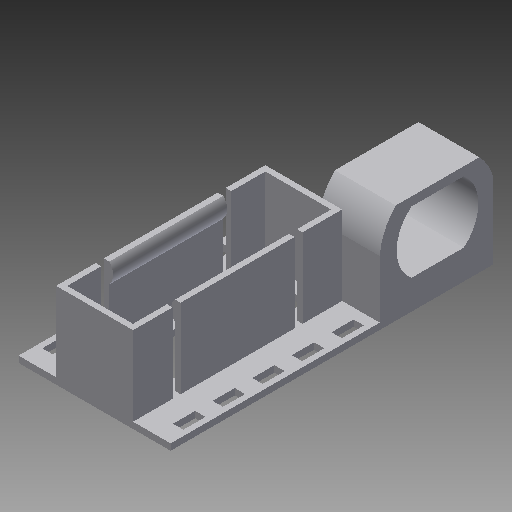
# Autodesk Inventor part: Correct Motor Housing
Saved by Autodesk Inventor 2018 (Build 220112000, 112)
## iProperties
Created: 2014-10-09
Part Number: Correct Motor Housing
Material: Generic
Document SubType Name: Modeling
Designer: Justin
Density: 1 g/cm^3
Appearance: Default(2)
Mass: 11.5799 g
Surface Area: 123.279 cm^2
Volume: 11.5799 cm^3
Author: Justin
Autodesk Inventor part; units mm, degrees
ref_plane "YZ Plane" through (0, 0, 0) normal (1, 0, 0) x (0, 1, 0)
ref_plane "XZ Plane" through (0, 0, 0) normal (0, 1, 0) x (-1, 0, 0)
ref_plane "XY Plane" through (0, 0, 0) normal (0, 0, 1) x (1, 0, 0)
sketch "Sketch1" plane through (0, 0, 0) normal (0, 1, 0) x (-1, 0, 0)
  line L0 (-19.2, 26.4) -> (19.2, 26.4)
  line L1 (19.2, 26.4) -> (19.2, -26.4)
  line L2 (10.8, -26.4) -> (-10.8, -26.4)
  line L3 (-19.2, -26.4) -> (-19.2, 26.4)
  line L4 (-19.2, 26.4) -> (19.2, -26.4) construction
  line L5 (19.2, 26.4) -> (-19.2, -26.4) construction
  line L6 (-5.3, 22) -> (5.3, 22)
  line L7 (5.3, 22) -> (5.3, -22)
  line L8 (5.3, -22) -> (-5.3, -22)
  line L9 (-5.3, -22) -> (-5.3, 22)
  line L10 (-5.3, 22) -> (5.3, -22) construction
  line L11 (5.3, 22) -> (-5.3, -22) construction
  line L12 (-10.8, -26.4) -> (-10.8, -55.1)
  line L13 (-10.8, -55.1) -> (-19.2, -55.1)
  line L14 (-19.2, -55.1) -> (-19.2, -26.4)
  line L15 (10.8, -26.4) -> (19.2, -26.4)
  point P0 (0, 0)
  point P1 (13.2741, -55.1)
  dimension "d4" = 10.6
  dimension "d5" = 44
  dimension "d37" = 8.4
  constraints: 32 end point, 5 parallel, 4 horizontal, 4 midpoint, 3 perpendicular, 1 point on line, 1 vertical
  measures "d4" distance of L7.end L8.end
  measures "d5" distance of L6.end L7.end
  measures "d37" distance between parallel lines of L14 L12
extrude "Extrusion1" add sketch "Sketch1" along normal blind 1.6
sketch "Sketch3" plane through (0, 1.6, 0) normal (0, 1, 0) x (1, 0, 0)
  line L0 (-5.3, 22) -> (5.3, 22) projected
  line L1 (5.3, -22) -> (-5.3, -22) projected
  line L2 (-19.2, -26.4) -> (19.2, -26.4) projected
  line L3 (10.8, 26.4) -> (-19.2, 26.4) projected
  line L4 (9.7, -26.4) -> (-9.7, -26.4)
  line L5 (-9.7, -26.4) -> (-9.7, 26.4)
  line L6 (-9.7, 26.4) -> (9.7, 26.4)
  line L7 (9.7, 26.4) -> (9.7, -26.4)
  line L8 (9.7, -26.4) -> (-9.7, 26.4) construction
  line L9 (-9.7, -26.4) -> (9.7, 26.4) construction
  line L10 (8.3, -25) -> (-8.3, -25)
  line L11 (-8.3, -25) -> (-8.3, 25)
  line L12 (-8.3, 25) -> (8.3, 25)
  line L13 (8.3, 25) -> (8.3, -25)
  line L14 (8.3, -25) -> (-8.3, 25) construction
  line L15 (-8.3, -25) -> (8.3, 25) construction
  line L16 (-9.7, 16.4) -> (-8.3, 16.4)
  line L17 (-9.7, 14.4) -> (-8.3, 14.4)
  line L18 (-9.7, -14.4) -> (-8.3, -14.4)
  line L19 (-9.7, -16.4) -> (-8.3, -16.4)
  line L20 (0, 22) -> (0, -22)
  line L21 (9.7, 16.4) -> (8.3, 16.4)
  line L22 (9.7, 14.4) -> (8.3, 14.4)
  line L23 (9.7, -14.4) -> (8.3, -14.4)
  line L24 (9.7, -16.4) -> (8.3, -16.4)
  line L25 (8.3, 16.4) -> (8.3, 14.4)
  line L26 (9.7, 16.4) -> (9.7, 14.4)
  line L27 (9.7, -14.4) -> (9.7, -16.4)
  line L28 (8.3, -14.4) -> (8.3, -16.4)
  point P0 (19.2, 26.4)
  point P1 (-10.8, 26.4)
  point P2 (0, 0)
  point P3 (0, 0)
  dimension "d8" = 19.4
  dimension "d9" = 1.4
  dimension "d10" = 1.4
  dimension "d11" = 2
  dimension "d12" = 10
  dimension "d13" = 2
  dimension "d14" = 10
  constraints: 50 end point, 9 point on line, 8 midpoint, 8 symmetric about line, 7 parallel, 5 perpendicular, 2 collinear, 2 horizontal
  measures "d8" distance of L5.end L6.end
  measures "d9" distance between parallel lines of L6 L12
  measures "d10" distance between parallel lines of L7 L13
  measures "d11" distance between parallel lines of L17 L16
  measures "d12" distance between parallel lines of L3 L16
  measures "d13" distance between parallel lines of L19 L18
  measures "d14" distance between parallel lines of L2 L19
extrude "Extrusion2" add sketch "Sketch3" along normal blind 20 contours L5 L19 L11 L10 L13 L24 L7 L2 | L5 L17 L11 L18 | L23 L13 L22 L7 | L5 L3 L7 L21 L13 L12 L11 L16
sketch "Sketch8" plane through (0, 1.6, 0) normal (0, 1, 0) x (1, 0, 0)
  line L0 (19.2, -26.4) -> (19.2, 55.1) projected
  line L1 (10.8, 55.1) -> (19.2, 55.1)
  line L2 (19.2, 55.1) -> (19.2, 26.4)
  line L3 (19.2, 26.4) -> (10.8, 26.4)
  line L4 (10.8, 26.4) -> (10.8, 55.1)
  point P0 (0, 0)
  constraints: 8 end point, 2 parallel, 1 horizontal, 1 perpendicular, 1 point on line
extrude "Extrusion6" add sketch "Sketch8" along normal blind 23.6
sketch "Sketch9" plane through (10.8, 0, -55.1) normal (-1, 0, 0) x (0, 0, 1)
  line L0 (28.7, 0) -> (0, 0) projected
  line L1 (28.7, 0) -> (28.7, 1.6) projected
  line L2 (28.7, 1.6) -> (28.7, 25.2) projected
  line L3 (0, 25.2) -> (28.7, 25.2) projected
  line L4 (0, 0) -> (0, 25.2) projected
  point P0 (55.1, 0)
extrude "Extrusion7" add sketch "Sketch9" along normal blind 7
sketch "Sketch10" plane through (19.2, 0, -55.1) normal (0, 0, -1) x (-1, 0, 0)
  line L0 (15.4, 0) -> (0, 0) projected
  line L1 (15.4, 25.2) -> (15.4, 0) projected
  line L2 (8.4, 0) -> (15.4, 7.2)
  point P0 (19.2, 0)
  dimension "d42" = 7.2
  dimension "d43" = 7
  constraints: 2 end point, 2 point on line
  measures "d42" distance of L0.start L2.end
  measures "d43" distance from line of L1 L2.start
extrude "Extrusion8" cut sketch "Sketch10" against normal up to surface (28.7 mm away)
sketch "Sketch11" plane through (19.2, 0, 26.4) normal (1, 0, 0) x (0, 0, -1)
  line L0 (81.5, 0) -> (0, 0) projected
  line L1 (81.5, 0) -> (81.5, 25.2) projected
  line L2 (52.8, 25.2) -> (81.5, 25.2) projected
  line L3 (52.8, 1.6) -> (52.8, 25.2) projected
  line L4 (52.8, 7.4) -> (81.5, 7.4)
  line L5 (55.0793, 23) -> (79.6991, 23)
  arc A0 (60.8, 23) -> (60.8, 7.4) centre (67.0851, 15.2) ccw
  arc A1 (74, 7.4) -> (74, 23) centre (67.6284, 15.2) ccw
  arc A2 (56.8391, 25.2) -> (52.8, 16.1566) centre (67.0851, 15.2) ccw
  line L6 (52.8, 14.2434) -> (52.8, 7.4)
  line L7 (52.8, 7.4) -> (60.8, 7.4)
  line L8 (74.3931, 7.4) -> (81.5, 7.4)
  arc A3 (81.5, 18.9579) -> (77.9504, 25.2) centre (67.6284, 15.2) ccw
  line L9 (81.5, 11.4421) -> (81.5, 7.4)
  line L10 (77.9504, 25.2) -> (56.8391, 25.2)
  arc A4 (56.8391, 25.2) -> (52.8, 16.1566) centre (67.0851, 15.2) ccw
  line L11 (56.8391, 25.2) -> (52.8, 25.2)
  line L12 (52.8, 25.2) -> (52.8, 14.2434)
  line L13 (77.9504, 25.2) -> (81.5, 25.2)
  line L14 (81.5, 25.2) -> (81.5, 18.9579)
  arc A5 (56.8391, 25.2) -> (52.8, 16.1566) centre (67.0851, 15.2) ccw
  line L15 (52.8, 16.1566) -> (52.8, 25.2)
  line L16 (52.8, 25.2) -> (56.8391, 25.2)
  point P0 (26.4, 0)
  point P1 (77.7, 15.2)
  point P2 (57.1, 15.2)
  dimension "d46" = 7.4
  dimension "d47" = 2.2
  dimension "d48" = 8
  dimension "d49" = 13.2
  dimension "d50" = 7.8
  dimension "d51" = 3.7
  dimension "d52" = 8
  dimension "d53" = 13.2
  dimension "d54" = 7.8
  dimension "d55" = 3.7
  dimension "d56" = 4.3
  dimension "d57" = 4.3
  constraints: 26 end point, 15 point on circle, 13 point on line, 6 centre point, 6 collinear, 5 perpendicular
  measures "d46" distance between parallel lines of L0 L4
  measures "d47" distance between parallel lines of L5 L2
  measures "d48" distance from line of A0.start L3
  measures "d49" distance of A0.start A1.end
  measures "d50" distance from line of L5 point (77.7, 15.2)
  measures "d51" horizontal distance of point (77.7, 15.2) A1.end
  measures "d52" distance from line of L3 L7.end
  measures "d53" distance of A1.start L7.end
  measures "d54" vertical distance of A0.start point (57.1, 15.2)
  measures "d55" horizontal distance of L7.end point (57.1, 15.2)
  measures "d56" radial gap between concentric circles of A2 A0
  measures "d57" radial gap between concentric circles of A3 A1
extrude "Extrusion9" cut sketch "Sketch11" against normal up to surface (15.4 mm away) contours A3 L2 L1 | L4 A0 L5 A1 | A2 L3 L2
sketch "Sketch12" plane through (0, 0, 0) normal (0, -1, 0) x (1, 0, 0)
  line L0 (19.2, -55.1) -> (19.2, 26.4) projected
  line L1 (19.2, 26.4) -> (-19.2, 26.4) projected
  line L2 (-5.3, 22) -> (5.3, 22) projected
  line L3 (5.3, -22) -> (-5.3, -22) projected
  line L4 (15.2, 21.8) -> (17.8, 21.8)
  line L5 (17.8, 21.8) -> (17.8, 16.2)
  line L6 (17.8, 16.2) -> (15.2, 16.2)
  line L7 (15.2, 16.2) -> (15.2, 21.8)
  line L8 (0, 22) -> (0, -22)
  line L9 (15.2, 11.8) -> (17.8, 11.8)
  line L10 (17.8, 11.8) -> (17.8, 6.2)
  line L11 (17.8, 6.2) -> (15.2, 6.2)
  line L12 (15.2, 6.2) -> (15.2, 11.8)
  line L13 (15.2, 1.8) -> (17.8, 1.8)
  line L14 (17.8, 1.8) -> (17.8, -3.8)
  line L15 (17.8, -3.8) -> (15.2, -3.8)
  line L16 (15.2, -3.8) -> (15.2, 1.8)
  line L17 (15.2, -8.2) -> (17.8, -8.2)
  line L18 (17.8, -8.2) -> (17.8, -13.8)
  line L19 (17.8, -13.8) -> (15.2, -13.8)
  line L20 (15.2, -13.8) -> (15.2, -8.2)
  line L21 (15.2, -18.2) -> (17.8, -18.2)
  line L22 (17.8, -18.2) -> (17.8, -23.8)
  line L23 (17.8, -23.8) -> (15.2, -23.8)
  line L24 (15.2, -23.8) -> (15.2, -18.2)
  line L25 (15.2, -28.2) -> (17.8, -28.2)
  line L26 (17.8, -28.2) -> (17.8, -33.8)
  line L27 (17.8, -33.8) -> (15.2, -33.8)
  line L28 (15.2, -33.8) -> (15.2, -28.2)
  line L29 (15.2, -38.2) -> (17.8, -38.2)
  line L30 (17.8, -38.2) -> (17.8, -43.8)
  line L31 (17.8, -43.8) -> (15.2, -43.8)
  line L32 (15.2, -43.8) -> (15.2, -38.2)
  line L33 (15.2, -48.2) -> (17.8, -48.2)
  line L34 (17.8, -48.2) -> (17.8, -53.8)
  line L35 (17.8, -53.8) -> (15.2, -53.8)
  line L36 (15.2, -53.8) -> (15.2, -48.2)
  line L37 (-15.2, 21.8) -> (-17.8, 21.8)
  line L38 (-17.8, 21.8) -> (-17.8, 16.2)
  line L39 (-17.8, 16.2) -> (-15.2, 16.2)
  line L40 (-15.2, 16.2) -> (-15.2, 21.8)
  line L41 (-15.2, 11.8) -> (-17.8, 11.8)
  line L42 (-17.8, 11.8) -> (-17.8, 6.2)
  line L43 (-15.2, 6.2) -> (-15.2, 11.8)
  line L44 (-17.8, 6.2) -> (-15.2, 6.2)
  line L45 (-15.2, 1.8) -> (-17.8, 1.8)
  line L46 (-17.8, 1.8) -> (-17.8, -3.8)
  line L47 (-15.2, -3.8) -> (-15.2, 1.8)
  line L48 (-17.8, -3.8) -> (-15.2, -3.8)
  line L49 (-15.2, -8.2) -> (-17.8, -8.2)
  line L50 (-17.8, -8.2) -> (-17.8, -13.8)
  line L51 (-15.2, -13.8) -> (-15.2, -8.2)
  line L52 (-17.8, -13.8) -> (-15.2, -13.8)
  line L53 (-15.2, -18.2) -> (-17.8, -18.2)
  line L54 (-17.8, -18.2) -> (-17.8, -23.8)
  line L55 (-15.2, -23.8) -> (-15.2, -18.2)
  line L56 (-17.8, -23.8) -> (-15.2, -23.8)
  point P0 (0, 0)
  dimension "d60" = 1.4
  dimension "d61" = 5.6
  dimension "d62" = 4.6
  dimension "d63" = 2.6
  dimension "d66" = 10
  constraints: 106 end point, 20 symmetric about line, 2 midpoint, 2 parallel, 1 horizontal, 1 perpendicular, 1 vertical, 56 other
  measures "d60" distance between parallel lines of L0 L5
  measures "d61" distance between parallel lines of L6 L4
  measures "d62" distance between parallel lines of L1 L4
  measures "d63" distance between parallel lines of L7 L5
  measures "d66" distance of L4.start L9.start
extrude "Extrusion10" cut sketch "Sketch12" against normal blind 5
sketch "Sketch13" plane through (8.3, 1.6, -14.4) normal (-1, 0, 0) x (0, 0, 1)
  line L0 (28.8, 0) -> (28.8, 20) projected
  line L1 (0, 20) -> (28.8, 20) projected
  line L2 (0, 20) -> (28.8, 20)
  line L3 (28.8, 20) -> (28.8, 15)
  line L4 (28.8, 15) -> (0, 15)
  line L5 (0, 15) -> (0, 20)
  point P0 (14.4, -1.6)
  dimension "d73" = 5
  constraints: 8 end point, 2 parallel, 1 horizontal, 1 perpendicular, 1 point on line
  measures "d73" distance between parallel lines of L4 L2
extrude "Extrusion11" add sketch "Sketch13" along normal blind 5
sketch "Sketch14" plane through (8.3, 1.6, 14.4) normal (0, 0, 1) x (1, 0, 0)
  line L0 (1.4, 20) -> (-5, 20) projected
  line L1 (-5, 15) -> (-5, 20) projected
  line L2 (0, 15) -> (-5, 15) projected
  line L3 (0, 15) -> (0, 20)
  arc A0 (0, 20) -> (0, 15) centre (2.625, 17.5) ccw
  point P0 (-8.3, -1.6)
  point P1 (-1, 17.5)
  dimension "d76" = 1
  constraints: 3 point on circle, 2 end point, 1 centre point, 1 perpendicular, 1 point on line
  measures "d76" distance from line of point (-1, 17.5) L3
extrude "Extrusion12" cut sketch "Sketch14" against normal up to surface (28.8 mm away) contours A0 L2 L1 L0
mirror "Mirror1" about plane through (0, 0, 0) normal (1, 0, 0) of "Extrusion11", "Extrusion12"
body "Solid1"
